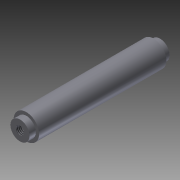
# Autodesk Inventor part: lower box weel shaft steel 2
Saved by Autodesk Inventor 2012 (Build 160160000, 160)
## iProperties
Created: 2012-12-28
Part Number: lower box weel shaft steel 2
Material: Default
Document SubType Name: Modeling
Designer: Bryce
Density: 1 g/cm^3
Author: Bryce
Autodesk Inventor part; units mm, degrees
ref_plane "YZ Plane" through (0, 0, 0) normal (1, 0, 0) x (0, 1, 0)
ref_plane "XZ Plane" through (0, 0, 0) normal (0, 1, 0) x (-1, 0, 0)
ref_plane "XY Plane" through (0, 0, 0) normal (0, 0, 1) x (1, 0, 0)
sketch "Sketch1" plane through (0, 0, 0) normal (0, 0, 1) x (1, 0, 0)
  circle A0 centre (0, 0) radius 6.35
  dimension "d0" = 12.7
  constraints: 1 centre point, 1 coincident
  measures "d0" diameter of A0
extrude "Extrusion1" add sketch "Sketch1" against normal blind 69.85
sketch "Sketch6" plane through (0, 0, 0) normal (0, 0, 1) x (1, 0, 0)
  circle A0 centre (0, 0) radius 6.35 projected
  circle A1 centre (0, 0) radius 2.0828
  circle A2 centre (0, 0) radius 4.7625
  dimension "d43" = 4.1656
  dimension "d44" = 9.525
  constraints: 2 centre point, 2 coincident
  measures "d43" diameter of A1
  measures "d44" diameter of A2
extrude "Extrusion11" cut sketch "Sketch6" against normal blind 3.175 contours A0
sketch "Sketch7" plane through (0, 0, -69.85) normal (0, 0, -1) x (-1, 0, 0)
  circle A0 centre (0, 0) radius 6.35 projected
  circle A1 centre (0, 0) radius 4.7625 projected
extrude "Extrusion12" cut sketch "Sketch7" against normal blind 3.175
extrude "Extrusion13" cut sketch "Sketch6" against normal through all contours A1
thread "Thread7" size "8-32 UNC" class "2B" standard "ANSI Unified Screw Threads" full length
body "Solid1"
